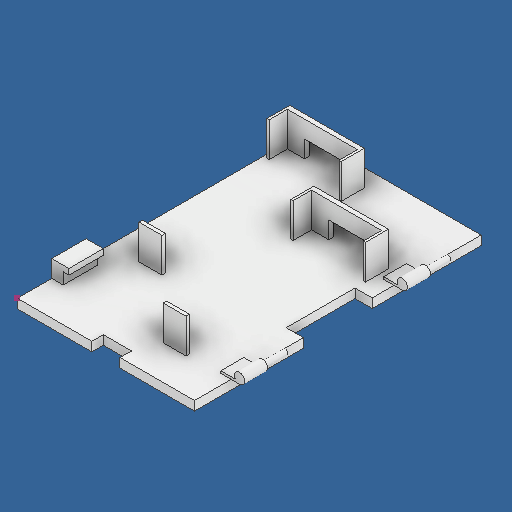
# Autodesk Inventor part: under plaque
Saved by Autodesk Inventor 2025 (Build 290162000, 162)
## iProperties
Created: 2024-08-14
Part Number: under plaque
Material: LCP Plastic
Document SubType Name: Modeling
Designer: Pauline Simonnet
Density: 1.626 g/cm^3
Appearance: Smooth - White
Author: Pauline Simonnet
Autodesk Inventor part; units mm, degrees
ref_plane "YZ Plane" through (0, 0, 0) normal (1, 0, 0) x (0, 1, 0)
ref_plane "XZ Plane" through (0, 0, 0) normal (0, 1, 0) x (-1, 0, 0)
ref_plane "XY Plane" through (0, 0, 0) normal (0, 0, 1) x (1, 0, 0)
sketch "Sketch1" plane through (0, 0, 0) normal (0, 1, 0) x (-1, 0, 0)
  line L0 (0, 0) -> (-154.5, 0)
  line L1 (-154.5, 0) -> (-154.5, -250)
  line L2 (-154.5, -250) -> (0, -250)
  line L3 (0, -250) -> (0, 0)
  dimension "d0" = 250
  dimension "d1" = 154.5
  constraints: 8 end point, 2 parallel, 1 horizontal, 1 perpendicular
  measures "d0" distance between parallel lines of L2 L0
  measures "d1" distance between parallel lines of L1 L3
extrude "Extrusion1" add sketch "Sketch1" along normal blind 8
sketch "Sketch2" plane through (0, 8, 0) normal (0, 1, 0) x (1, 0, 0)
  line L0 (154.5, 0) -> (154.5, 250) construction
  line L1 (154.5, 195) -> (145.5, 195) construction
  line L2 (145.5, 195) -> (145.5, 215) construction
  line L3 (145.5, 215) -> (154.5, 215) construction
  line L4 (154.5, 215) -> (154.5, 195) construction
  line L5 (154.5, 53) -> (145.5, 53) construction
  line L6 (145.5, 53) -> (145.5, 73) construction
  line L7 (145.5, 73) -> (154.5, 73) construction
  line L8 (154.5, 73) -> (154.5, 53) construction
  line L9 (154.5, 250) -> (0, 250) construction
  line L10 (0, 0) -> (154.5, 0) construction
  line L11 (145.5, 32) -> (163.8, 32)
  line L12 (163.8, 32) -> (163.8, 52)
  line L13 (163.8, 52) -> (145.5, 52)
  line L14 (145.5, 52) -> (145.5, 32)
  line L15 (145.5, 174) -> (163.8, 174)
  line L16 (163.8, 174) -> (163.8, 194)
  line L17 (163.8, 194) -> (145.5, 194)
  line L18 (145.5, 194) -> (145.5, 174)
  dimension "d4" = 35
  dimension "d6" = 20
  dimension "d7" = 20
  dimension "d8" = 9
  dimension "d9" = 20
  dimension "d10" = 1
  dimension "d11" = 1
  dimension "d12" = 20
  dimension "d13" = 9.3
  dimension "d14" = 9
  dimension "d15" = 9.3
  dimension "d16" = 9
  dimension "d142" = 32
  constraints: 32 end point, 8 parallel, 4 horizontal, 4 perpendicular, 3 point on line
  measures "d4" distance between parallel lines of L9 L3
  measures "d6" distance between parallel lines of L7 L5
  measures "d7" distance between parallel lines of L3 L1
  measures "d8" distance between parallel lines of L0 L6
  measures "d9" distance between parallel lines of L13 L11
  measures "d10" distance between parallel lines of L5 L13
  measures "d11" distance between parallel lines of L1 L17
  measures "d12" distance between parallel lines of L17 L15
  measures "d13" distance between parallel lines of L12 L0
  measures "d14" distance between parallel lines of L0 L14
  measures "d15" distance between parallel lines of L16 L0
  measures "d16" distance between parallel lines of L0 L18
  measures "d142" distance between parallel lines of L11 L10
extrude "Extrusion2" add sketch "Sketch2" along normal blind 2
sketch "Sketch3" plane through (154.5, 8, -32) normal (0, 0, 1) x (1, 0, 0)
  circle A0 centre (7.3, 4.5) radius 4.5
  line L0 (-9, 2) -> (9.3, 2) projected
  line L1 (9.3, 0) -> (9.3, 2) projected
  line L2 (0, 0) -> (9.3, 0) projected
  point P0 (-154.5, -8)
  point P1 (3.6382, 1.8844)
  point P2 (10.9618, 1.8844)
  point P3 (9.3, 0.4689)
  point P4 (3.5583, 2)
  point P5 (7.3, 0)
  dimension "d20" = 9
  dimension "d22" = 2
  dimension "d30" = 4.5
  constraints: 2 point on circle, 1 centre point
  measures "d20" diameter of A0
  measures "d22" distance from line of L1 A0.centre
  measures "d30" distance from line of A0.centre L2
extrude "Extrusion3" add sketch "Sketch3" against normal blind 20 contours A0 L1 L0 | L0 L1 A0
sketch "Sketch4" plane through (154.5, 8, -32) normal (0, 0, 1) x (1, 0, 0)
  circle A0 centre (7.3, 4.5) radius 2.125
  arc A1 (9.3, 0.4689) -> (3.5583, 2) centre (7.3, 4.5) ccw projected
  point P0 (-154.5, -8)
  dimension "d25" = 4.25
  dimension "d26" = 0
  dimension "d27" = 0
  constraints: 1 centre point
  measures "d25" diameter of A0
  measures "d26" distance of A1.centre A0.centre
  measures "d27" distance of A1.centre A0.centre
extrude "Extrusion4" add sketch "Sketch4" against normal blind 40
fillet "Fillet1" radius 9 1 edges at (163.8, 8, -42)
sketch "Sketch5" plane through (154.5, 8, -174) normal (0, 0, 1) x (1, 0, 0)
  circle A0 centre (7.3, 4.5) radius 4.5
  line L0 (0, 0) -> (9.3, 0) projected
  line L1 (9.3, 0) -> (9.3, 2) projected
  point P0 (-154.5, -8)
  dimension "d32" = 4.5
  dimension "d33" = 9
  dimension "d34" = 2
  constraints: 1 centre point
  measures "d32" distance from line of A0.centre L0
  measures "d33" diameter of A0
  measures "d34" distance from line of L1 A0.centre
extrude "Extrusion5" add sketch "Sketch5" against normal blind 20 contours A0
sketch "Sketch6" plane through (154.5, 8, -174) normal (0, 0, 1) x (1, 0, 0)
  circle A0 centre (7.3, 4.5) radius 2.125
  arc A1 (9.3, 0.4689) -> (3.5583, 2) centre (7.3, 4.5) ccw projected
  point P0 (-154.5, -8)
  dimension "d37" = 4.25
  dimension "d38" = 0
  dimension "d39" = 0
  constraints: 1 centre point
  measures "d37" diameter of A0
  measures "d38" distance of A1.centre A0.centre
  measures "d39" distance of A0.centre A1.centre
extrude "Extrusion6" add sketch "Sketch6" against normal blind 40
fillet "Fillet2" radius 9 1 edges at (163.8, 8, -184)
sketch "Sketch7" plane through (0, 8, 0) normal (0, 1, 0) x (1, 0, 0)
  point P0 (0, 0)
sketch "Sketch8" plane through (0, 8, 0) normal (0, 1, 0) x (1, 0, 0)
  line L0 (154.5, 52) -> (154.5, 174) projected
  line L1 (139.5, 95) -> (154.5, 95)
  line L2 (154.5, 95) -> (154.5, 155)
  line L3 (154.5, 155) -> (139.5, 155)
  line L4 (139.5, 155) -> (139.5, 95)
  line L5 (0, 0) -> (154.5, 0) projected
  line L6 (65, 0) -> (89.5, 0)
  line L7 (89.5, 0) -> (89.5, 10)
  line L8 (89.5, 10) -> (65, 10)
  line L9 (65, 10) -> (65, 0)
  line L10 (0, 250) -> (0, 0) projected
  line L11 (154.5, 0) -> (154.5, 32) projected
  line L12 (154.5, 250) -> (0, 250) projected
  point P0 (89.5, 0)
  dimension "d43" = 65
  dimension "d44" = 65
  dimension "d45" = 10
  dimension "d46" = 95
  dimension "d47" = 95
  dimension "d48" = 15
  constraints: 16 end point, 4 parallel, 2 horizontal, 2 perpendicular, 2 point on line
  measures "d43" distance between parallel lines of L9 L10
  measures "d44" distance between parallel lines of L7 L11
  measures "d45" distance between parallel lines of L8 L5
  measures "d46" distance between parallel lines of L1 L5
  measures "d47" distance between parallel lines of L12 L3
  measures "d48" distance between parallel lines of L2 L4
extrude "Extrusion7" cut sketch "Sketch8" against normal through all
sketch "Sketch9" plane through (0, 8, 0) normal (0, 1, 0) x (1, 0, 0)
  line L0 (139.6215, 164) -> (139.6215, 184)
  line L1 (139.6215, 184) -> (137.6215, 184)
  line L2 (137.6215, 184) -> (137.6215, 164)
  line L3 (137.6215, 164) -> (139.6215, 164)
  line L4 (139.6215, 180) -> (139.6215, 184)
  line L5 (139.6215, 184) -> (74.6215, 184)
  line L6 (74.6215, 184) -> (74.6215, 180)
  line L7 (74.6215, 180) -> (139.6215, 180)
  line L8 (74.6215, 184) -> (74.6215, 164)
  line L9 (74.6215, 164) -> (76.6215, 164)
  line L10 (76.6215, 164) -> (76.6215, 184)
  line L11 (76.6215, 184) -> (74.6215, 184)
  line L12 (154.5, 250) -> (0, 250) projected
  line L13 (0, 250) -> (0, 0) projected
  line L14 (68.0244, 214.5619) -> (68.0244, 234.5619)
  line L15 (68.0244, 234.5619) -> (66.0244, 234.5619)
  line L16 (66.0244, 234.5619) -> (66.0244, 214.5619)
  line L17 (66.0244, 214.5619) -> (68.0244, 214.5619)
  line L18 (3.0244, 214.5619) -> (5.0244, 214.5619)
  line L19 (5.0244, 214.5619) -> (5.0244, 234.5619)
  line L20 (3.0244, 234.5619) -> (3.0244, 214.5619)
  line L21 (3.0244, 234.5619) -> (3.0244, 230.5619)
  line L22 (5.0244, 234.5619) -> (3.0244, 234.5619)
  line L23 (3.0244, 230.5619) -> (68.0244, 230.5619)
  line L24 (68.0244, 234.5619) -> (3.0244, 234.5619)
  line L25 (68.0244, 230.5619) -> (68.0244, 234.5619)
  line L26 (25.5244, 83.5619) -> (45.5244, 83.5619)
  line L27 (45.5244, 83.5619) -> (45.5244, 80.5619)
  line L28 (45.5244, 80.5619) -> (25.5244, 80.5619)
  line L29 (25.5244, 80.5619) -> (25.5244, 83.5619)
  line L30 (97.1215, 33) -> (117.1215, 33)
  line L31 (117.1215, 33) -> (117.1215, 30)
  line L32 (117.1215, 30) -> (97.1215, 30)
  line L33 (97.1215, 30) -> (97.1215, 33)
  point P0 (137.6215, 180)
  point P1 (76.6215, 180)
  point P2 (5.0244, 230.5619)
  point P3 (66.0244, 230.5619)
  dimension "d65" = 2
  dimension "d66" = 2
  dimension "d69" = 61
  dimension "d77" = 20
  dimension "d109" = 2
  dimension "d110" = 2
  dimension "d113" = 61
  dimension "d120" = 20
  dimension "d143" = 147
  dimension "d144" = 3
  dimension "d145" = 20
  dimension "d146" = 20.5
  dimension "d147" = 20.5
  dimension "d148" = 147
  dimension "d149" = 20.5
  dimension "d150" = 3
  dimension "d151" = 20
  constraints: 64 end point, 16 parallel, 8 perpendicular, 6 point on line, 2 horizontal
  measures "d65" distance between parallel lines of L2 L0
  measures "d66" distance between parallel lines of L8 L10
  measures "d69" distance between parallel lines of L10 L2
  measures "d77" distance between parallel lines of L11 L9
  measures "d109" distance between parallel lines of L16 L14
  measures "d110" distance between parallel lines of L20 L19
  measures "d113" distance between parallel lines of L19 L16
  measures "d120" distance between parallel lines of L22 L18
  measures "d143" distance between parallel lines of L26 L23
  measures "d144" distance between parallel lines of L28 L26
  measures "d145" distance between parallel lines of L27 L29
  measures "d146" distance between parallel lines of L29 L19
  measures "d147" distance between parallel lines of L16 L27
  measures "d148" distance between parallel lines of L30 L7
  measures "d149" distance between parallel lines of L33 L10
  measures "d150" distance between parallel lines of L32 L30
  measures "d151" distance between parallel lines of L31 L33
extrude "Extrusion8" add sketch "Sketch9" along normal blind 30
sketch "Sketch13" plane through (5.0244, 8, -230.5619) normal (0, 0, 1) x (1, 0, 0)
  line L0 (-2, 0) -> (63, 0) projected
  line L1 (15, 0) -> (46, 0)
  line L2 (46, 0) -> (46, 15)
  line L3 (46, 15) -> (15, 15)
  line L4 (15, 15) -> (15, 0)
  line L5 (61, 0) -> (61, 30) projected
  line L6 (0, 30) -> (61, 30) projected
  line L7 (0, 0) -> (0, 30) projected
  point P0 (-5.0244, -8)
  dimension "d124" = 15
  dimension "d125" = 15
  dimension "d126" = 15
  constraints: 8 end point, 2 parallel, 1 horizontal, 1 perpendicular, 1 point on line
  measures "d124" distance between parallel lines of L5 L2
  measures "d125" distance between parallel lines of L3 L6
  measures "d126" distance between parallel lines of L4 L7
extrude "Extrusion12" cut sketch "Sketch13" against normal blind 30 contours L4 L3 L2 L0
sketch "Sketch14" plane through (76.6215, 8, -180) normal (0, 0, 1) x (1, 0, 0)
  line L0 (-2, 0) -> (63, 0) projected
  line L1 (15, 0) -> (46, 0)
  line L2 (46, 0) -> (46, 15)
  line L3 (46, 15) -> (15, 15)
  line L4 (15, 15) -> (15, 0)
  line L5 (61, 0) -> (61, 30) projected
  line L6 (0, 30) -> (61, 30) projected
  line L7 (0, 0) -> (0, 30) projected
  point P0 (-76.6215, -8)
  dimension "d129" = 15
  dimension "d130" = 15
  dimension "d131" = 15
  constraints: 8 end point, 2 parallel, 1 horizontal, 1 perpendicular, 1 point on line
  measures "d129" distance between parallel lines of L5 L2
  measures "d130" distance between parallel lines of L3 L6
  measures "d131" distance between parallel lines of L4 L7
extrude "Extrusion13" cut sketch "Sketch14" against normal blind 30 contours L4 L3 L2 L0
sketch "Sketch15" plane through (0, 8, 0) normal (0, 1, 0) x (1, 0, 0)
  line L0 (0, 250) -> (0, 0) projected
  line L1 (0, 60) -> (10, 60)
  line L2 (10, 60) -> (10, 30)
  line L3 (10, 30) -> (0, 30)
  line L4 (0, 30) -> (0, 60)
  line L5 (0, 0) -> (65, 0) projected
  point P0 (5, 30)
  point P1 (5, 60)
  point P2 (0, 30)
  dimension "d134" = 30
  dimension "d135" = 30
  dimension "d136" = 10
  constraints: 8 end point, 2 midpoint, 2 parallel, 1 horizontal, 1 perpendicular, 1 point on line
  measures "d134" distance from line of L5 point (5, 30)
  measures "d135" distance of point (5, 30) point (5, 60)
  measures "d136" distance between parallel lines of L2 L0
extrude "Extrusion14" add sketch "Sketch15" along normal blind 15
sketch "Sketch16" plane through (10, 8, -30) normal (1, 0, 0) x (0, 0, -1)
  line L0 (0, 0) -> (0, 15) projected
  line L1 (30, 0) -> (30, 15) projected
  line L2 (0, 15) -> (30, 15)
  line L3 (30, 15) -> (30, 10)
  line L4 (30, 10) -> (0, 10)
  line L5 (0, 10) -> (0, 15)
  point P0 (-30, -8)
  point P1 (0, 10)
  dimension "d139" = 5
  constraints: 8 end point, 2 parallel, 1 horizontal, 1 perpendicular, 1 point on line
  measures "d139" distance between parallel lines of L4 L2
extrude "Extrusion15" add sketch "Sketch16" along normal blind 5
equation "\"d15\" = d13"
body "Solid1"
